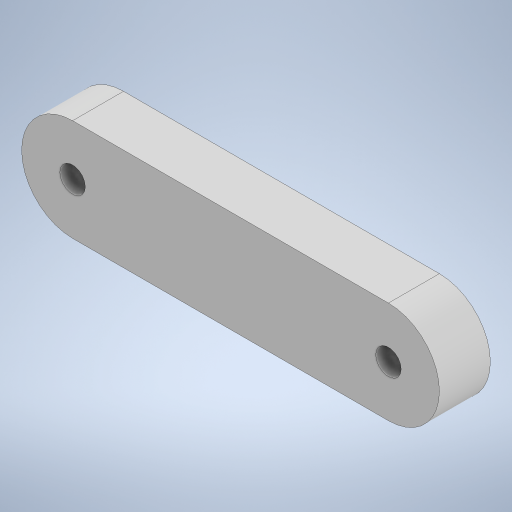
# Autodesk Inventor part: bunny tendon
Saved by Autodesk Inventor 2024.2 (Build 282272000, 272)
## iProperties
Created: 2025-12-17
Part Number: bunny tendon
Material: Generic
Document SubType Name: Modeling
Designer: David Toler II
Density: 1 g/cm^3
Appearance: Default
Author: David Toler II
Autodesk Inventor part; units mm, degrees
ref_plane "YZ Plane" through (0, 0, 0) normal (1, 0, 0) x (0, 1, 0)
ref_plane "XZ Plane" through (0, 0, 0) normal (0, 1, 0) x (-1, 0, 0)
ref_plane "XY Plane" through (0, 0, 0) normal (0, 0, 1) x (1, 0, 0)
sketch "Sketch1" plane through (0, 0, 0) normal (0, 0, 1) x (1, 0, 0)
  line L0 (19.685, 0) -> (-19.685, 0) construction
  line L1 (19.685, 6.35) -> (-19.685, 6.35)
  line L2 (-19.685, -6.35) -> (19.685, -6.35)
  arc A0 (19.685, -6.35) -> (19.685, 6.35) centre (19.685, 0) ccw
  arc A1 (-19.685, 6.35) -> (-19.685, -6.35) centre (-19.685, 0) ccw
  circle A2 centre (-19.685, 0) radius 1.5875
  circle A3 centre (19.685, 0) radius 1.5875
  point P0 (0, 0)
  dimension "d0" = 6.35
  dimension "d1" = 3.175
  dimension "d2" = 3.175
  dimension "d3" = 39.37
  constraints: 8 end point, 4 centre point, 4 point on circle, 4 tangent, 2 coincident, 1 horizontal, 1 midpoint, 1 parallel
  measures "d0" radius of A1
  measures "d1" diameter of A2
  measures "d2" diameter of A3
  measures "d3" distance of L0.start L0.end
extrude "Extrusion1" add sketch "Sketch1" along normal blind 6.35
body "Solid1"
